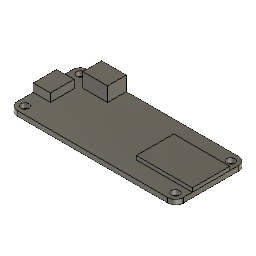
3010 Feather M0 Wifi (Autodesk Fusion 360 design; units mm, degrees)
Autodesk Fusion 360 part; units mm, degrees
sketch "board" plane through (0, 0, 0) normal (0, 0, 1) x (1, 0, 0)
  line L0 (0, 0) -> (53.34, 0)
  line L1 (53.34, 0) -> (53.34, 22.86)
  line L2 (53.34, 22.86) -> (0, 22.86)
  line L3 (0, 22.86) -> (0, 0)
  circle A0 centre (2.54, 20.32) radius 1.27
  circle A1 centre (50.8, 20.32) radius 1.27
  circle A2 centre (2.54, 2.54) radius 1.27
  circle A3 centre (50.8, 2.54) radius 1.27
  dimension "d1" = 53.34
  dimension "d2" = 22.86
  dimension "d3" = 2.54
  dimension "d4" = 2.54
  dimension "d5" = 2.54
  dimension "d8" = 48.26
  dimension "d9" = -17.78
  measures "d1" distance of L1.end L2.end
  measures "d2" distance of L0.start L2.end
  measures "d3" diameter of A0
  measures "d4" distance of L3 A0.centre
  measures "d5" distance of L2 A0.centre
extrude "Extrude1" add sketch "board" along normal blind 1.6 makes body 1
fillet "Fillet1" radius 2.54 4 edges at (0, 22.86, 0.8) (0, 0, 0.8) (53.34, 22.86, 0.8) (53.34, 0, 0.8) on bodies 1
sketch "usb" plane through (0, 0, 1.6) normal (0, 0, 1) x (-1, 0, 0)
  circle A0 centre (-50.8, -20.32) radius 1.27
  circle A1 centre (-50.8, -2.54) radius 1.27
  circle A2 centre (-2.54, -2.54) radius 1.27
  circle A3 centre (-2.54, -20.32) radius 1.27
  arc A4 (-50.8, 0) -> (-53.34, -2.54) centre (-50.8, -2.54) ccw
  line L0 (-53.34, -2.54) -> (-53.34, -20.32)
  arc A5 (-53.34, -20.32) -> (-50.8, -22.86) centre (-50.8, -20.32) ccw
  line L1 (-50.8, -22.86) -> (-2.54, -22.86)
  arc A6 (-2.54, -22.86) -> (0, -20.32) centre (-2.54, -20.32) ccw
  line L2 (0, -20.32) -> (0, -2.54)
  arc A7 (0, -2.54) -> (-2.54, 0) centre (-2.54, -2.54) ccw
  line L3 (-2.54, 0) -> (-50.8, 0)
  line L4 (0, -11.43) -> (-53.34, -11.43) construction
  line L5 (-26.67, -22.86) -> (-26.67, 0) construction
  line L6 (0, -15.23) -> (-5.6, -15.23)
  line L7 (-5.6, -15.23) -> (-5.6, -7.63)
  line L8 (-5.6, -7.63) -> (0, -7.63)
  line L9 (0, -7.63) -> (0, -15.23)
  line L10 (0, -11.43) -> (-5.6, -11.43) construction
  dimension "d13" = 7.6
  dimension "d14" = 5.6
  measures "d13" distance of L6.start L8.end
  measures "d14" distance of L6.start L6.end
extrude "Extrude2" add sketch "usb" along normal blind 2.6 separate body contours L2 L6 L7 L8 L9 makes body 2
sketch "jst" plane through (0, 0, 1.6) normal (0, 0, 1) x (-1, 0, 0)
  circle A0 centre (-50.8, -20.32) radius 1.27
  circle A1 centre (-50.8, -2.54) radius 1.27
  circle A2 centre (-2.54, -2.54) radius 1.27
  circle A3 centre (-2.54, -20.32) radius 1.27
  arc A4 (-50.8, 0) -> (-53.34, -2.54) centre (-50.8, -2.54) ccw
  line L0 (-53.34, -2.54) -> (-53.34, -20.32)
  arc A5 (-53.34, -20.32) -> (-50.8, -22.86) centre (-50.8, -20.32) ccw
  line L1 (-50.8, -22.86) -> (-2.54, -22.86)
  arc A6 (-2.54, -22.86) -> (0, -20.32) centre (-2.54, -20.32) ccw
  line L2 (0, -20.32) -> (0, -2.54)
  arc A7 (0, -2.54) -> (-2.54, 0) centre (-2.54, -2.54) ccw
  line L3 (-2.54, 0) -> (-50.8, 0)
  line L4 (-6.8, -22.86) -> (-14.8, -22.86)
  line L5 (-14.8, -22.86) -> (-14.8, -16.76)
  line L6 (-14.8, -16.76) -> (-6.8, -16.76)
  line L7 (-6.8, -16.76) -> (-6.8, -22.86)
  dimension "d17" = 6.1
  dimension "d18" = 8
  dimension "d19" = 6.8
  measures "d17" distance of L4.start L6.end
  measures "d18" distance of L4.start L4.end
  measures "d19" distance of L2 L7
extrude "Extrude3" add sketch "jst" along normal blind 4.6 separate body contours L1 L4 L5 L6 L7 makes body 3
sketch "wifi" plane through (0, 0, 1.6) normal (0, 0, 1) x (-1, 0, 0)
  circle A0 centre (-50.8, -20.32) radius 1.27
  circle A1 centre (-50.8, -2.54) radius 1.27
  circle A2 centre (-2.54, -2.54) radius 1.27
  circle A3 centre (-2.54, -20.32) radius 1.27
  arc A4 (-50.8, 0) -> (-53.34, -2.54) centre (-50.8, -2.54) ccw
  line L0 (-53.34, -2.54) -> (-53.34, -20.32)
  arc A5 (-53.34, -20.32) -> (-50.8, -22.86) centre (-50.8, -20.32) ccw
  line L1 (-50.8, -22.86) -> (-2.54, -22.86)
  arc A6 (-2.54, -22.86) -> (0, -20.32) centre (-2.54, -20.32) ccw
  line L2 (0, -20.32) -> (0, -2.54)
  arc A7 (0, -2.54) -> (-2.54, 0) centre (-2.54, -2.54) ccw
  line L3 (-2.54, 0) -> (-50.8, 0)
  line L4 (-35.34, -17.43) -> (-53.34, -17.43)
  line L5 (-53.34, -17.43) -> (-53.34, -5.43)
  line L6 (-53.34, -5.43) -> (-35.34, -5.43)
  line L7 (-35.34, -5.43) -> (-35.34, -17.43)
  line L8 (-35.34, -11.43) -> (-53.34, -11.43) construction
  line L9 (-53.34, -11.43) -> (0, -11.43) construction
  dimension "d22" = 18
  dimension "d23" = 12
  measures "d22" distance of L4.start L4.end
  measures "d23" distance of L4.end L5.end
extrude "Extrude4" add sketch "wifi" along normal blind 1.2 separate body contours L0 L4 L5 L6 L7 makes body 4
sketch "Sketch1" plane through (0, 0, 0) normal (0, 0, -1) x (1, 0, 0) in component "board tester"
  arc A0 (53.34, -2.54) -> (50.8, 0) centre (50.8, -2.54) ccw construction
  line L0 (50.8, 0) -> (2.54, 0)
  arc A1 (2.54, 0) -> (0, -2.54) centre (2.54, -2.54) ccw construction
  line L1 (0, -2.54) -> (0, -20.32) construction
  arc A2 (0, -20.32) -> (2.54, -22.86) centre (2.54, -20.32) ccw
  line L2 (2.54, -22.86) -> (50.8, -22.86)
  arc A3 (50.8, -22.86) -> (53.34, -20.32) centre (50.8, -20.32) ccw
  line L3 (53.34, -20.32) -> (53.34, -2.54) construction
  circle A4 centre (50.8, -20.32) radius 1.27
  circle A5 centre (50.8, -2.54) radius 1.27 construction
  circle A6 centre (2.54, -2.54) radius 1.27
  circle A7 centre (2.54, -20.32) radius 1.27
  circle A8 centre (50.8, -2.54) radius 2.9
  circle A9 centre (50.8, -2.54) radius 1.4
  circle A10 centre (2.54, -2.54) radius 1.4
  circle A11 centre (2.54, -2.54) radius 2.9
  circle A12 centre (50.8, -20.32) radius 1.4
  circle A13 centre (50.8, -20.32) radius 2.9
  circle A14 centre (2.54, -20.32) radius 1.4
  circle A15 centre (2.54, -20.32) radius 2.9
  line L4 (26.67, -22.86) -> (26.67, 0) construction
  line L5 (0, -11.43) -> (53.34, -11.43) construction
  line L6 (-2.46, -25.32) -> (55.8, -25.32)
  line L7 (55.8, -25.32) -> (55.8, 2.46)
  line L8 (55.8, 2.46) -> (-2.46, 2.46)
  line L9 (-2.46, 2.46) -> (-2.46, -25.32)
  line L10 (-2.46, -25.32) -> (55.8, 2.46) construction
  line L11 (55.8, -25.32) -> (-2.46, 2.46) construction
  line L12 (6.67, -18.43) -> (46.67, -18.43)
  line L13 (46.67, -18.43) -> (46.67, -4.43)
  line L14 (46.67, -4.43) -> (6.67, -4.43)
  line L15 (6.67, -4.43) -> (6.67, -18.43)
  line L16 (6.67, -18.43) -> (46.67, -4.43) construction
  line L17 (46.67, -18.43) -> (6.67, -4.43) construction
  point P0 (26.67, -11.43)
  point P1 (26.67, -11.43)
  dimension "d27" = 2.8
  dimension "d28" = 1.5
  dimension "d31" = -48.26
  dimension "d32" = -17.78
  dimension "d33" = 5
  dimension "d34" = 5
  dimension "d35" = 40
  dimension "d36" = 14
  measures "d27" diameter of A9
  measures "d28" distance of A8 A9
  measures "d33" distance of A2.centre L6
  measures "d34" distance of A2.centre L9
  measures "d35" distance of L13.end L14.end
  measures "d36" distance of L12.end L13.end
extrude "Extrude1'" add sketch "Sketch1" along normal blind 5 and the other way blind -4 separate body contours A8 | A11 | A13 | A15 | L6 L7 L8 L9 makes body 5 in component "board tester"
extrude "Extrude2'" add sketch "Sketch1" along normal blind 5 and the other way blind 0 contours A8 | A11 | A13 | A15 bodies 5 in component "board tester"
fillet "Fillet1'" radius 3 4 edges at (-2.46, -2.46, -4.5) (-2.46, 25.32, -4.5) (55.8, 25.32, -4.5) (55.8, -2.46, -4.5) on bodies 5 in component "board tester"
component "board tester" placed x (1, 0, 0) y (0, 1, 0) z (0, 0, 1) at (0, 0, 0)
named bodies: "board", "microUSB", "JST connector", "WiFI Chip", "moun tester"
